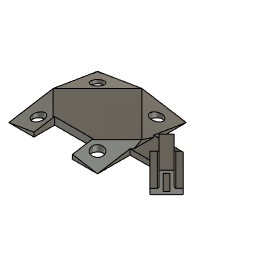
pinsfacingdown (Autodesk Fusion 360 design; units mm, degrees)
Autodesk Fusion 360 part; units mm, degrees
sketch "Sketch1" plane through (0, 0, 0) normal (0, 0, 1) x (1, 0, 0)
  line L0 (-15, -15) -> (15, -15)
  line L1 (15, -15) -> (15, 15)
  line L2 (15, 15) -> (-15, 15)
  line L3 (-15, 15) -> (-15, -15)
  line L4 (-15, -15) -> (15, 15) construction
  line L5 (15, -15) -> (-15, 15) construction
  dimension "d1" = 30
  dimension "d2" = 30
  constraint horizontal L0
  constraint perpendicular L0 L1
  constraint parallel L0 L2
  constraint parallel L1 L3
  constraint coincident L4 origin
  constraint coincident L5 origin
  measures "d1" distance of L1.end L2.end
  measures "d2" distance of L0.end L1.end
extrude "Extrude1" add sketch "Sketch1" along normal blind 5 makes body 1
ref_plane "WorkPlane1" through (-15, -15, 0) normal (-0.162221, -0.162221, 0.973329) x (0.707107, -0.707107, 0)
sketch "Sketch2" plane through (-15, -15, 0) normal (-0.162221, -0.162221, 0.973329) x (0.707107, -0.707107, 0)
  line L0 (-26, 0) -> (26, 0)
  line L1 (26, 0) -> (26, 44)
  line L2 (26, 44) -> (-26, 44)
  line L3 (-26, 44) -> (-26, 0)
  line L4 (-26, 0) -> (26, 44) construction
  line L5 (26, 0) -> (-26, 44) construction
  point P0 (0, 22)
  constraint horizontal L0
  constraint perpendicular L0 L1
  constraint parallel L0 L2
  constraint parallel L1 L3
  constraint coincident L4 P0
  constraint coincident L5 P0
extrude "Extrude2" cut sketch "Sketch2" along normal blind 3 bodies 1 makes body 2 at (-5, 5, 0)
ref_plane "WorkPlane2" through (-15, 15, 0) normal (-0.162221, 0.162221, 0.973329) x (-0.707107, -0.707107, 0)
sketch "Sketch3" plane through (-15, 15, 0) normal (-0.162221, 0.162221, 0.973329) x (-0.707107, -0.707107, 0)
  line L0 (-24.7973, -1.8328) -> (24.7973, -1.8328)
  line L1 (24.7973, -1.8328) -> (24.7973, 45.8328)
  line L2 (24.7973, 45.8328) -> (-24.7973, 45.8328)
  line L3 (-24.7973, 45.8328) -> (-24.7973, -1.8328)
  line L4 (-24.7973, -1.8328) -> (24.7973, 45.8328) construction
  line L5 (24.7973, -1.8328) -> (-24.7973, 45.8328) construction
  point P0 (0, 22)
  constraint horizontal L0
  constraint perpendicular L0 L1
  constraint parallel L0 L2
  constraint parallel L1 L3
  constraint coincident L4 P0
  constraint coincident L5 P0
extrude "Extrude3" cut sketch "Sketch3" along normal blind 3 bodies 1 2 makes body 3 at (-5, 5, 0)
ref_plane "WorkPlane3" through (15, 15, 0) normal (0.162221, 0.162221, 0.973329) x (-0.707107, 0.707107, 0)
sketch "Sketch4" plane through (15, 15, 0) normal (0.162221, 0.162221, 0.973329) x (-0.707107, 0.707107, 0)
  line L0 (-26.4896, -3.4019) -> (26.4896, -3.4019)
  line L1 (26.4896, -3.4019) -> (26.4896, 47.4019)
  line L2 (26.4896, 47.4019) -> (-26.4896, 47.4019)
  line L3 (-26.4896, 47.4019) -> (-26.4896, -3.4019)
  line L4 (-26.4896, -3.4019) -> (26.4896, 47.4019) construction
  line L5 (26.4896, -3.4019) -> (-26.4896, 47.4019) construction
  point P0 (0, 22)
  constraint horizontal L0
  constraint perpendicular L0 L1
  constraint parallel L0 L2
  constraint parallel L1 L3
  constraint coincident L4 P0
  constraint coincident L5 P0
extrude "Extrude4" cut sketch "Sketch4" along normal blind 3 bodies 2 3 makes body 4 at (-5, 5, 0)
ref_plane "WorkPlane4" through (15, -15, 0) normal (0.162221, -0.162221, 0.973329) x (0.707107, 0.707107, 0)
sketch "Sketch5" plane through (15, -15, 0) normal (0.162221, -0.162221, 0.973329) x (0.707107, 0.707107, 0)
  line L0 (-20.5685, -0.9126) -> (20.5685, -0.9126)
  line L1 (20.5685, -0.9126) -> (20.5685, 44.9126)
  line L2 (20.5685, 44.9126) -> (-20.5685, 44.9126)
  line L3 (-20.5685, 44.9126) -> (-20.5685, -0.9126)
  line L4 (-20.5685, -0.9126) -> (20.5685, 44.9126) construction
  line L5 (20.5685, -0.9126) -> (-20.5685, 44.9126) construction
  point P0 (0, 22)
  constraint horizontal L0
  constraint perpendicular L0 L1
  constraint parallel L0 L2
  constraint parallel L1 L3
  constraint coincident L4 P0
  constraint coincident L5 P0
extrude "Extrude5" cut sketch "Sketch5" along normal blind 3 bodies 1 3 4 makes body 5 at (-5, 5, 0)
extrude "Extrude6" cut 1 faces at (-5, 5, 3.3333) along direction (-0.162221, 0.162221, 0.973329) blind 6 on bodies 5 bodies 2
extrude "Extrude7" cut 1 faces at (-5, -5, 3.3333) along direction (-0.162221, -0.162221, 0.973329) blind 5 on bodies 5 bodies 1
extrude "Extrude8" cut 1 faces at (10, -10, 1.6667) along direction (0.162221, -0.162221, 0.973329) blind 5 on bodies 5 bodies 4
extrude "Extrude9" cut 1 faces at (10, 10, 1.6667) along direction (0.162221, 0.162221, 0.973329) blind 5 on bodies 5 bodies 3
sketch "Sketch6" plane through (0, 0, 0) normal (0, 0, -1) x (1, 0, 0)
  line L0 (-15, 15) -> (-15, -15)
  line L1 (-15, -15) -> (15, -15)
  line L2 (15, -15) -> (15, 15)
  line L3 (15, 15) -> (-15, 15)
  line L4 (10, 10) -> (-10, 10)
  line L5 (-10, 10) -> (-10, -10)
  line L6 (-10, -10) -> (10, -10)
  line L7 (10, -10) -> (10, 10)
  line L8 (10, 10) -> (-10, -10) construction
  line L9 (-10, 10) -> (10, -10) construction
  circle A0 centre (-10, 10) radius 2
  circle A1 centre (10, 10) radius 2
  circle A2 centre (-10, -10) radius 2
  circle A3 centre (10, -10) radius 2
  dimension "d21" = 20
  dimension "d22" = 20
  dimension "d23" = 4
  dimension "d24" = 4
  dimension "d25" = 4
  dimension "d26" = 4
  constraint horizontal L4
  constraint perpendicular L4 L5
  constraint parallel L4 L6
  constraint parallel L5 L7
  constraint coincident L8 origin
  constraint coincident L9 origin
  constraint coincident L4.end L5.start
  constraint coincident L4.start L7.end
  constraint coincident L5.end L6.start
  constraint coincident L6.end L7.start
  measures "d21" distance of L5.end L6.end
  measures "d22" distance of L4.end L5.end
  measures "d23" diameter of A0
  measures "d24" diameter of A1
  measures "d25" diameter of A2
  measures "d26" diameter of A3
extrude "Extrude10" cut sketch "Sketch6" against normal blind 5 contours L4 L5 A0 | L4 L5 A0 | L4 L7 A1 | L4 L7 A1 | L5 L6 A2 | L5 L6 A2 | L6 L7 A3 | L6 L7 A3 bodies 5
sketch "Sketch7" plane through (0, 0, 0) normal (0, 0, -1) x (1, 0, 0)
  circle A0 centre (-10, -10) radius 2
  circle A1 centre (-10, 10) radius 2
  circle A2 centre (10, -10) radius 2
  circle A3 centre (10, 10) radius 2
  line L0 (-15, 15) -> (-15, -15)
  line L1 (-15, -15) -> (15, -15)
  line L2 (15, -15) -> (15, 15)
  line L3 (15, 15) -> (-15, 15)
  line L4 (-6.5, -8) -> (6.5, -8)
  line L5 (6.5, -8) -> (6.5, 8)
  line L6 (6.5, 8) -> (-6.5, 8)
  line L7 (-6.5, 8) -> (-6.5, -8)
  line L8 (-6.5, -8) -> (6.5, 8) construction
  line L9 (6.5, -8) -> (-6.5, 8) construction
  line L10 (-6.5, 8) -> (6.5, 8)
  line L11 (6.5, 8) -> (6.5, 12)
  line L12 (6.5, 12) -> (-6.5, 12)
  line L13 (-6.5, 12) -> (-6.5, 8)
  dimension "d29" = 13
  dimension "d30" = 16
  dimension "d31" = 13
  dimension "d32" = 4
  constraint horizontal L4
  constraint perpendicular L4 L5
  constraint parallel L4 L6
  constraint parallel L5 L7
  constraint coincident L8 origin
  constraint coincident L9 origin
  constraint horizontal L10
  constraint vertical L11
  constraint horizontal L12
  constraint vertical L13
  measures "d29" distance of L5.end L6.end
  measures "d30" distance of L4.end L5.end
  measures "d31" distance of L6.end L5.end
  measures "d32" distance of L6.end L12.end
extrude "Extrude11" cut sketch "Sketch7" against normal blind 5 contours L6 L10 L11 L12 L13 bodies 5
sketch "Sketch8" plane through (0, -15, 0) normal (0, -1, 0) x (1, 0, 0)
  line L0 (15, 0) -> (0, 2.5)
  line L1 (0, 2.5) -> (-15, 0)
  line L2 (-15, 0) -> (15, 0)
  line L3 (6.5, 1) -> (-6.5, 1)
  line L4 (-6.5, 1) -> (-6.5, -1)
  line L5 (-6.5, -1) -> (6.5, -1)
  line L6 (6.5, -1) -> (6.5, 1)
  line L7 (6.5, 1) -> (-6.5, -1) construction
  line L8 (-6.5, 1) -> (6.5, -1) construction
  line L9 (-6.5, 1) -> (6.5, 1)
  line L10 (6.5, 1) -> (6.5, 5.3332)
  line L11 (6.5, 5.3332) -> (-6.5, 5.3332)
  line L12 (-6.5, 5.3332) -> (-6.5, 1)
  dimension "d35" = 13
  dimension "d36" = 2
  dimension "d37" = 13
  constraint horizontal L3
  constraint perpendicular L3 L4
  constraint parallel L3 L5
  constraint parallel L4 L6
  constraint coincident L7 origin
  constraint coincident L8 origin
  constraint horizontal L9
  constraint vertical L10
  constraint horizontal L11
  constraint vertical L12
  measures "d35" distance of L4.end L5.end
  measures "d36" distance of L3.end L4.end
  measures "d37" distance of L3.end L3.start
extrude "Extrude12" cut sketch "Sketch8" against normal blind 5 contours L0 L1 L3 L9 L10 L12 | L0 L1 L10 L11 L12 bodies 5
sketch "Sketch9" plane through (-15, 0, 0) normal (-1, 0, 0) x (0, -1, 0)
  line L0 (0, 2.5) -> (-15, 0)
  line L1 (-15, 0) -> (15, 0)
  line L2 (15, 0) -> (0, 2.5)
  line L3 (0, 2.5) -> (-15, 2.5)
  line L4 (-15, 2.5) -> (-15, 5.5)
  line L5 (-15, 5.5) -> (0, 5.5)
  line L6 (0, 5.5) -> (0, 2.5)
  line L7 (0, 2.5) -> (15, 2.5)
  line L8 (15, 2.5) -> (15, 5.5)
  line L9 (15, 5.5) -> (0, 5.5)
  line L10 (0, 5.5) -> (0, 2.5)
  dimension "d41" = 15
  dimension "d42" = 3
  dimension "d43" = 3
  constraint horizontal L3
  constraint vertical L4
  constraint horizontal L5
  constraint vertical L6
  constraint coincident L0.start L2.end
  constraint horizontal L7
  constraint vertical L8
  constraint horizontal L9
  constraint vertical L10
  measures "d41" distance of L0.start L3.end
  measures "d42" distance of L0.start L5.end
  measures "d43" distance of L0.start L5.end
extrude "Extrude13" cut sketch "Sketch9" against normal blind 30 contours L3 L4 L5 L6 L10 | L6 L7 L8 L9 L10 bodies 5
extrude "Extrude14" cut sketch "Sketch8" against normal blind 5 contours L2 L3 L4 L6 L9 bodies 5
sketch "Sketch10" plane through (15, 0, 0) normal (1, 0, 0) x (0, 1, 0)
  line L0 (0, 2.5) -> (-15, 0)
  line L1 (-15, 0) -> (15, 0)
  line L2 (15, 0) -> (0, 2.5)
  line L3 (0, 0) -> (4, 0)
  line L4 (4, 0) -> (4, 1.8333)
  line L5 (-4, 1.8333) -> (-4, 0)
  line L6 (0, 0) -> (-4, 0)
  line L7 (-4, 1.8333) -> (4, 1.8333)
  dimension "d48" = 4
  constraint coincident L3.start L6.start
  constraint parallel L1 L3
  constraint coincident L2 L4.end
  constraint perpendicular L1 L4
  constraint coincident L0 L5.start
  constraint coincident L1 L5.end
  constraint perpendicular L1 L5
  constraint perpendicular L4 L7
  measures "d48" distance of L3.start L3.end
extrude "Extrude15" add sketch "Sketch10" along normal blind 10 contours L1 L3 L4 L5 L6 L7 bodies 1 2 3 4 5
ref_plane "WorkPlane5" through (25, 4, 0.9167) normal (-0.707107, 0.707107, 0) x (0, 0, 1)
sketch "Sketch11" plane through (25, 4, 0.9167) normal (-0.707107, 0.707107, 0) x (0, 0, 1)
  line L0 (0, 0) -> (0.918, 0)
  line L1 (0.918, 0) -> (0.918, -8)
  line L2 (0.918, -8) -> (-0.917, -8)
  line L3 (-0.917, -8) -> (-0.917, 0)
  line L4 (0, 0) -> (-0.917, 0)
  dimension "d52" = 0.918
  dimension "d53" = 8
  dimension "d54" = 1.835
  constraint coincident L0.start L4.start
  constraint horizontal L0
  constraint perpendicular L0 L1
  constraint perpendicular L1 L2
  constraint perpendicular L2 L3
  constraint perpendicular L3 L4
  measures "d52" distance of L0.start L0.end
  measures "d53" distance of L0.end L1.end
  measures "d54" distance of L1.end L2.end
extrude "Extrude16" add sketch "Sketch11" against normal blind 15 bodies 1
sketch "Sketch15" plane through (21.1066, -21.1066, 0) normal (0.707107, -0.707107, 0) x (0.707107, 0.707107, 0)
  line L0 (20.5061, -0.0003) -> (20.5061, 1.8347)
  line L1 (20.5061, 1.8347) -> (12.5061, 1.8347)
  line L2 (12.5061, 1.8347) -> (12.5061, -0.0003)
  line L3 (12.5061, -0.0003) -> (20.5061, -0.0003)
  line L4 (14.7061, 7.1347) -> (18.3061, 7.1347)
  line L5 (18.3061, 7.1347) -> (18.3061, -3.4653)
  line L6 (18.3061, -3.4653) -> (14.7061, -3.4653)
  line L7 (14.7061, -3.4653) -> (14.7061, 7.1347)
  line L8 (14.7061, 7.1347) -> (18.3061, -3.4653) construction
  line L9 (18.3061, 7.1347) -> (14.7061, -3.4653) construction
  line L10 (14.7061, 0.7886) -> (18.3061, 0.7886)
  line L11 (18.3061, 0.7886) -> (18.3061, 7.1347)
  line L12 (18.3061, 7.1347) -> (14.7061, 7.1347)
  line L13 (14.7061, 7.1347) -> (14.7061, 0.7886)
  point P0 (16.5061, 1.8347)
  dimension "d65" = 3.6
  dimension "d66" = 10.6
  constraint horizontal L4
  constraint perpendicular L4 L5
  constraint parallel L4 L6
  constraint parallel L5 L7
  constraint coincident L8 P0
  constraint coincident L9 P0
  constraint midpoint L1 P0
  constraint horizontal L10
  constraint vertical L11
  constraint horizontal L12
  constraint vertical L13
  constraint coincident L7 L10.start
  measures "d65" distance of L5.end L6.end
  measures "d66" distance of L4.end L5.end
extrude "Extrude19" add sketch "Sketch15" against normal blind 15 contours L1 L5 L7 L10 L11 L13 | L1 L4 L5 L7 L11 L12 L13 bodies 1
sketch "Sketch16" plane through (21.1066, -21.1066, 0) normal (0.707107, -0.707107, 0) x (0.707107, 0.707107, 0)
  line L0 (14.7061, 1.8347) -> (12.5061, 1.8347)
  line L1 (12.5061, 1.8347) -> (12.5061, -0.0003)
  line L2 (12.5061, -0.0003) -> (20.5061, -0.0003)
  line L3 (20.5061, -0.0003) -> (20.5061, 1.8347)
  line L4 (20.5061, 1.8347) -> (18.3061, 1.8347)
  line L5 (18.3061, 1.8347) -> (18.3061, 7.1347)
  line L6 (18.3061, 7.1347) -> (14.7061, 7.1347)
  line L7 (14.7061, 7.1347) -> (14.7061, 1.8347)
  line L8 (16.5061, -0.0003) -> (16.5061, 7.1347)
  line L9 (15.7061, 6.2172) -> (17.3061, 6.2172)
  line L10 (17.3061, 6.2172) -> (17.3061, 0.9172)
  line L11 (17.3061, 0.9172) -> (15.7061, 0.9172)
  line L12 (15.7061, 0.9172) -> (15.7061, 6.2172)
  line L13 (15.7061, 6.2172) -> (17.3061, 0.9172) construction
  line L14 (17.3061, 6.2172) -> (15.7061, 0.9172) construction
  point P0 (16.5061, 3.5672)
  dimension "d69" = 1.6
  dimension "d70" = 5.3
  constraint midpoint L2 L8.start
  constraint midpoint L6 L8.end
  constraint horizontal L9
  constraint perpendicular L9 L10
  constraint parallel L9 L11
  constraint parallel L10 L12
  constraint coincident L13 P0
  constraint coincident L14 P0
  constraint midpoint L8 P0
  measures "d69" distance of L10.end L11.end
  measures "d70" distance of L9.end L10.end
extrude "Extrude20" cut sketch "Sketch16" against normal blind 14 contours L8 L9 L10 L11 | L8 L9 L11 L12 bodies 1
chamfer "Chamfer1" distance 0.66 angle 45 1 edges at (15, 0, 1.8333) on bodies 1
chamfer "Chamfer2" distance 0.4 angle 45 2 edges at (26.2021, -5.4045, 1.8347) (28.7477, -2.8589, 1.8347) on bodies 1
chamfer "Chamfer2" distance 0.4 angle 45 1 edges at (22.1716, 1.1716, 1.8333) on bodies 1
